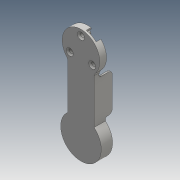
# Autodesk Inventor part: proteção celula de carga Rafa-
Saved by Autodesk Inventor 2016 (Build 200138000, 138)
## iProperties
Created: 2017-10-16
Part Number: proteção celula de carga Rafa-
Material: Generic
Document SubType Name: Modeling
Designer: Ascânio
Density: 1 g/cm^3
Appearance: Default
Author: Ascânio
Autodesk Inventor part; units mm, degrees
ref_plane "YZ Plane" through (0, 0, 0) normal (1, 0, 0) x (0, 1, 0)
ref_plane "XZ Plane" through (0, 0, 0) normal (0, 1, 0) x (-1, 0, 0)
ref_plane "XY Plane" through (0, 0, 0) normal (0, 0, 1) x (1, 0, 0)
sketch "Sketch1" plane through (0, 0, 0) normal (0, 1, 0) x (-1, 0, 0)
  circle A0 centre (0, 0) radius 25
  line L0 (17.5, 0) -> (-17.5, 0)
  line L1 (-17.5, 0) -> (-17.5, -75)
  line L2 (-17.5, -75) -> (17.5, -75)
  line L3 (17.5, -75) -> (17.5, 0)
  circle A1 centre (0, -100) radius 27
  line L4 (-17.5, -75) -> (-17.5, -100)
  line L5 (-17.5, -100) -> (17.5, -100)
  line L6 (17.5, -100) -> (17.5, -75)
  dimension "d0" = 50
  dimension "d1" = 35
  dimension "d2" = 17.5
  dimension "d4" = 75
  dimension "d49" = 54
  dimension "d60" = 0
  dimension "d61" = 25
  constraints: 14 end point, 2 centre point, 2 midpoint, 2 parallel, 2 perpendicular, 1 coincident, 1 collinear, 1 horizontal, 1 vertical
  measures "d0" diameter of A0
  measures "d1" distance of L1.end L2.end
  measures "d2" distance from line of point (0, 0) L3
  measures "d4" distance from line of L2 A0.centre
  measures "d49" diameter of A1
  measures "d60" horizontal distance of A1.centre point (0, 0)
  measures "d61" distance from line of A1.centre L2
extrude "Extrusion1" add sketch "Sketch1" along normal blind 2
sketch "Sketch2" plane through (0, 2, 0) normal (0, 1, 0) x (1, 0, 0)
  arc A0 (-17.5, 17.8536) -> (17.5, 17.8536) centre (0, 0) ccw projected
  line L0 (-17.5, 79.4391) -> (-17.5, 17.8536) projected
  line L1 (17.5, 17.8536) -> (17.5, 79.4391) projected
  circle A1 centre (-14.9389, 8.625) radius 4.35
  circle A2 centre (14.9389, 8.625) radius 4.35
  circle A3 centre (0, -17.25) radius 4.35
  line L2 (-14.9389, 8.625) -> (14.9389, 8.625) construction
  line L3 (14.9389, 8.625) -> (0, -17.25) construction
  line L4 (0, -17.25) -> (-14.9389, 8.625) construction
  line L5 (-14.9389, 8.625) -> (0, 0) construction
  line L6 (0, 0) -> (14.9389, 8.625) construction
  line L7 (0, -17.25) -> (0, 0) construction
  arc A4 (17.5, 79.4391) -> (-17.5, 79.4391) centre (0, 100) ccw projected
  line L8 (15.5, 80.385) -> (15.5, 16.9926)
  arc A5 (-15.5, 16.9926) -> (15.5, 16.9926) centre (0, 0) ccw
  line L9 (-15.5, 16.9926) -> (-15.5, 80.385)
  arc A6 (15.5, 80.385) -> (-15.5, 80.385) centre (0, 100) ccw
  circle A7 centre (0, 0) radius 17.25 construction
  point P0 (-17.5, 75)
  point P1 (17.5, 75)
  dimension "d8" = 8.7
  dimension "d9" = 8.7
  dimension "d10" = 8.7
  dimension "d50" = 2
  dimension "d51" = 34.5
  dimension "d68" = 29.8779
  constraints: 16 end point, 6 centre point, 6 point on circle, 4 equal length, 1 point on line, 1 vertical, 3 other
  measures "d8" diameter of A1
  measures "d9" diameter of A2
  measures "d10" diameter of A3
  measures "d50" distance between parallel lines of L1 L8
  measures "d51" diameter of A7
  measures "d68" distance of L2.start L2.end
extrude "Extrusion2" add sketch "Sketch2" along normal blind 7
sketch "Sketch3" plane through (-14.9389, 9, -8.625) normal (0, 1, 0) x (1, 0, 0)
  circle A0 centre (0, 0) radius 2.65
  circle A1 centre (14.9389, -25.875) radius 4.35 projected
  circle A2 centre (14.9389, -25.875) radius 2.65
  circle A3 centre (29.8779, 0) radius 2.65
  circle A4 centre (0, 0) radius 4.35 projected
  circle A5 centre (29.8779, 0) radius 4.35 projected
  point P0 (14.9389, -8.625)
  dimension "d16" = 5.3
  constraints: 3 centre point, 2 concentric, 2 equal radius, 1 coincident
  measures "d16" diameter of A2
extrude "Extrusion3" cut sketch "Sketch3" against normal through all contours A0 | A2 | A3
chamfer "Chamfer1" distance 2 angle 45 3 edges at (-2.65, 0, 17.25) (12.2889, 0, -8.625) (-17.5889, 0, -8.625) measured on face at (5.8333, 0, -38.3821)
sketch "Sketch4" plane through (0, 0, 0) normal (0, 0, 1) x (1, 0, 0)
  line L0 (25, 9) -> (-25, 9) projected
  line L1 (23, 2) -> (-23, 2) projected
  line L2 (17.35, 9) -> (4.35, 9)
  line L3 (4.35, 9) -> (-4.35, 9) projected
  line L4 (-4.35, 2) -> (4.35, 2) projected
  line L5 (4.35, 2) -> (4.35, 9) projected
  line L6 (17.5, 9) -> (17.5, 2.675)
  line L7 (17.5, 2.675) -> (4.35, 2.675)
  line L8 (4.35, 9) -> (4.35, 2.675)
  point P0 (0, 0)
  point P1 (-17.5, 9)
  point P2 (-15.5, 2)
  point P3 (15.5, 2)
  dimension "d26" = 6.325
  constraints: 8 end point, 2 point on line, 1 collinear, 1 horizontal, 1 parallel, 1 perpendicular
  measures "d26" distance between parallel lines of L0 L7
extrude "Extrusion4" cut sketch "Sketch4" along normal through all
sketch "Sketch5" plane through (0, 9, 0) normal (0, 1, 0) x (1, 0, 0)
  line L0 (17.5, 75) -> (15.5, 75)
  line L1 (15.5, 75) -> (15.5, 25)
  line L2 (15.5, 25) -> (17.5, 25)
  line L3 (17.5, 25) -> (17.5, 75)
  line L4 (-17.5, 79.4391) -> (-17.5, 17.8536) projected
  line L5 (-15.5, 75) -> (-17.5, 75)
  line L6 (-17.5, 75) -> (-17.5, 25)
  line L7 (-17.5, 25) -> (-15.5, 25)
  line L8 (-15.5, 25) -> (-15.5, 75)
  line L9 (-15.5, 16.9926) -> (-15.5, 80.385) projected
  line L10 (15.5, 80.385) -> (15.5, 16.9926) projected
  line L11 (17.5, 17.8536) -> (17.5, 79.4391) projected
  point P0 (0, 0)
  dimension "d28" = 50
  dimension "d52" = 25
  constraints: 16 end point, 4 parallel, 3 collinear, 2 horizontal, 2 perpendicular, 2 point on line
  measures "d28" distance of L2.end L0.start
  measures "d52" distance from line of point (0, 0) L2
extrude "Extrusion5" add sketch "Sketch5" along normal blind 15
fillet "Fillet1" radius 5 2 edges at (17.5, 4.5, -17.8536) (-17.5, 4.5, -17.8536)
fillet "Fillet3" radius 5 4 edges at (-16.5, 24, -25) (16.5, 24, -25) (-16.5, 24, -75) (16.5, 24, -75)
sketch "Sketch7" plane through (-17.5, 0, -75) normal (-1, 0, 0) x (0, 0, 1)
  line L0 (53, 6) -> (60, 9)
  line L1 (60, 9) -> (53, 9)
  line L2 (53, 9) -> (53, 6)
  line L3 (50, 9) -> (55.1569, 9) projected
  line L4 (0, 9) -> (0, 19) projected
  line L5 (53, 9) -> (50, 9)
  line L6 (50, 9) -> (50, 6)
  line L7 (50, 6) -> (53, 6)
  line L8 (53, 6) -> (53, 9)
  line L9 (50, 9) -> (50, 19) projected
  point P0 (75, 0)
  point P1 (53, 9)
  point P2 (0, 0)
  point P3 (0, 2)
  dimension "d36" = 3
  dimension "d37" = 7
  dimension "d39" = 60
  constraints: 14 end point, 2 collinear, 2 parallel, 2 perpendicular, 1 horizontal
  measures "d36" distance of L1.end L0.start
  measures "d37" distance of L0.end L1.end
  measures "d39" distance from line of L4 L0.end
extrude "Extrusion6" cut sketch "Sketch7" along normal through all both and the other way through all
fillet "Fillet5" radius 3 2 edges at (-16.5, 6, -25) (16.5, 6, -25)
sketch "Sketch9" plane through (0, 2, 0) normal (0, 1, 0) x (1, 0, 0)
  circle A0 centre (0, 100) radius 20.5
  arc A1 (15.5, 80.385) -> (-15.5, 80.385) centre (0, 100) ccw projected
  circle A2 centre (0, 100) radius 17.5
  circle A3 centre (0, 100) radius 10
  circle A4 centre (0, 100) radius 7
  point P0 (0, 0)
  dimension "d53" = 3
  dimension "d54" = 35
  dimension "d55" = 3
  dimension "d56" = 20
  constraints: 4 centre point, 3 coincident, 1 concentric
  measures "d53" radial gap between concentric circles of A0 A2
  measures "d54" diameter of A2
  measures "d55" radial gap between concentric circles of A4 A3
  measures "d56" diameter of A3
extrude "Extrusion8" add sketch "Sketch9" along normal blind 3
sketch "Sketch10" plane through (0, 9, 0) normal (0, 1, 0) x (1, 0, 0)
  line L0 (17.5, 75) -> (17.5, 79.4391) projected
  arc A0 (17.5, 79.4391) -> (-17.5, 79.4391) centre (0, 100) ccw projected
  line L1 (-17.5, 79.4391) -> (-17.5, 75) projected
  line L2 (-15.5, 75) -> (-15.5, 80.385) projected
  arc A1 (15.5, 80.385) -> (-15.5, 80.385) centre (0, 100) ccw projected
  line L3 (15.5, 80.385) -> (15.5, 75) projected
  line L4 (17.5, 75) -> (15.5, 75) projected
  line L5 (-15.5, 75) -> (-17.5, 75) projected
  point P0 (0, 0)
extrude "Extrusion9" add sketch "Sketch10" along normal blind 6
fillet "Fillet7" radius 2 2 edges at (16.5, 15, -75) (-16.5, 15, -75)
body "Solid1"
